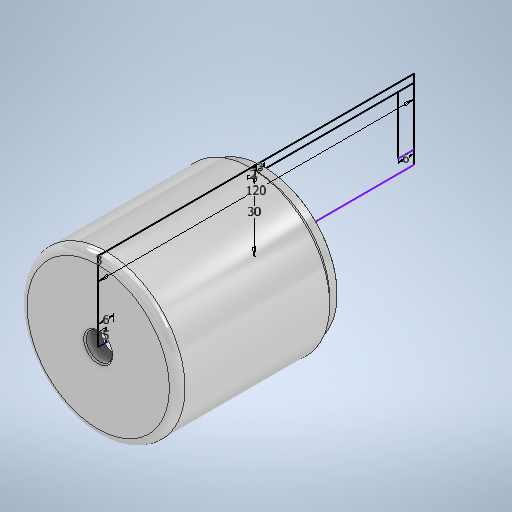
# Autodesk Inventor part: Plenum
Saved by Autodesk Inventor 2025.2 (Build 292293000, 293)
## iProperties
Created: 2026-06-25
Part Number: Plenum
Material: Generic
Document SubType Name: Modeling
Designer: Simon
Density: 1 g/cm^3
Appearance: Aluminum - Polished
Author: Simon
Autodesk Inventor part; units mm, degrees
ref_plane "YZ Plane" through (0, 0, 0) normal (1, 0, 0) x (0, 1, 0)
ref_plane "XZ Plane" through (0, 0, 0) normal (0, 1, 0) x (-1, 0, 0)
ref_plane "XY Plane" through (0, 0, 0) normal (0, 0, 1) x (1, 0, 0)
sketch "Sketch2" plane through (0, 0, 0) normal (1, 0, 0) x (0, 1, 0)
  line L0 (0, 0) -> (30, 0)
  line L1 (30, 60) -> (30, -60)
  line L2 (30, 60) -> (27, 60)
  line L3 (27, 60) -> (27, -60)
  line L4 (27, -60) -> (30, -60)
  line L5 (27, 60) -> (0, 60)
  line L6 (0, 60) -> (5, 60)
  line L7 (5, 60) -> (5, 54)
  line L8 (5, 54) -> (27, 54)
  line L9 (27, -60) -> (0, -60)
  line L10 (0, -60) -> (5, -60)
  line L11 (5, -60) -> (5, -54)
  line L12 (5, -54) -> (27, -54)
  line L13 (0, 60) -> (0, -60)
  line L14 (27, 0) -> (28, 0)
  line L15 (28, 0) -> (28, -3)
  line L16 (28, -3) -> (27, -3)
  line L17 (28, 0) -> (28, 2)
  line L18 (28, 2) -> (30, 2)
  line L19 (30, 2) -> (28, 0)
  dimension "d12" = 30
  dimension "d13" = 120
  dimension "d14" = 3
  dimension "d15" = 5
  dimension "d16" = 6
  dimension "d17" = 6
  dimension "d26" = 1
  dimension "d27" = 3
  dimension "d28" = 2
  constraints: 40 end point, 12 point on line, 7 perpendicular, 2 horizontal, 2 midpoint, 2 vertical, 1 parallel
  measures "d12" distance of L0.start L0.end
  measures "d13" distance of L1.start L1.end
  measures "d14" distance of L1.start L2.end
  measures "d15" distance of L5.end L6.end
  measures "d16" distance of L6.end L7.end
  measures "d17" distance of L10.end L11.end
  measures "d26" distance of L14.start L14.end
  measures "d27" distance of L14.end L15.end
  measures "d28" distance of L14.end L17.end
revolve "Revolution1" add sketch "Sketch2" angle 360 about axis through (0, 0, 60) along (0, 0, -1) contours L3 L2 L1 L18 L17 L0 | L0 L15 L16 L3 | L17 L18 L19 | L8 L7 L5 L3
fillet "Fillet2" radius 3 1 edges at (0, -30, 60)
thread "Thread3" size "M10x1.5" class "6H" standard "ISO Metric profile" full length
chamfer "Chamfer2" distance 0.5 angle 45 1 edges at (0, -5, 60)
fillet "Fillet3" radius 3 1 edges at (0, -27, 54)
chamfer "Chamfer3" distance 0.2 angle 45 1 edges at (0, -28, -3)
body "Solid2"
